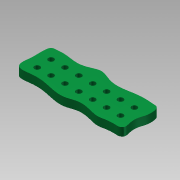
# Autodesk Inventor part: PBD-14 плата
Saved by Autodesk Inventor 2011 (Build 150239000, 239)
## iProperties
Created: 2011-01-23
Part Number: PBD-14 плата
Document SubType Name: Modeling
Designer: Aleirim
Density: 1 g/cm^3
Author: Aleirim
Autodesk Inventor part; units mm, degrees
ref_plane "YZ Plane" through (0, 0, 0) normal (1, 0, 0) x (0, 1, 0)
ref_plane "XZ Plane" through (0, 0, 0) normal (0, 1, 0) x (-1, 0, 0)
ref_plane "XY Plane" through (0, 0, 0) normal (0, 0, 1) x (1, 0, 0)
sketch "Эскиз1" plane through (0, 0, 0) normal (0, 0, 1) x (1, 0, 0)
  spline S0 degree 5 poles (-7.2879, -2.8745) (-6.5517, -2.7913) (-5.2414, -2.7026) (-3.2703, -3.1942) (0.1838, -4.3916) (1.2148, -1.7819) (5.9591, -4.1296) (5.9445, -3.1102) (9.2498, -3.1073) (8.9071, -3.3129) (10.262, -2.8139) (9.4235, -1.6551) (9.4476, 0.385) (10.1818, 0.941) (9.962, 3.5245) (9.2903, 3.5819) (8.0786, 3.5357) (5.6303, 4.053) (1.0268, 1.8567) (-1.261, 5.8579) (-3.117, 2.0115) (-7.1177, 3.7745) (-8.1331, 3.183) (-9.395, 3.43) (-9.6839, 2.8201) (-9.7254, 2.1391) (-9.7847, 0.8422) (-9.6013, -0.2797) (-10.1279, -1.9544) (-9.626, -3.1181) (-8.6028, -3.0516) (-7.7999, -2.9323) (-7.2879, -2.8745) knots 0 0 0 0 0 0 0.061225 0.101586 0.149698 0.194246 0.231169 0.262878 0.289475 0.316265 0.343376 0.374776 0.406255 0.437302 0.468259 0.504653 0.543723 0.588673 0.638889 0.687231 0.727539 0.761442 0.789632 0.813664 0.838456 0.866069 0.896043 0.929673 0.957419 1 1 1 1 1 1
  line L0 (-7.7526, -1.17) -> (-7.7526, -1.37) projected
  line L1 (-7.4863, -1.37) -> (-7.7526, -1.37) projected
  line L2 (-7.4863, -1.37) -> (-7.4863, -1.17) projected
  line L3 (-7.7526, -1.17) -> (-7.4863, -1.17) projected
  circle A0 centre (-7.6194, -1.27) radius 0.5
  line L4 (-7.6194, -1.37) -> (-7.6194, -1.17) construction
  line L5 (-7.7526, -1.27) -> (-7.4863, -1.27) construction
  circle A1 centre (-5.0794, -1.27) radius 0.5
  circle A2 centre (-2.5394, -1.27) radius 0.5
  circle A3 centre (0.0006, -1.27) radius 0.5
  circle A4 centre (2.5406, -1.27) radius 0.5
  circle A5 centre (5.0806, -1.27) radius 0.5
  circle A6 centre (7.6206, -1.27) radius 0.5
  circle A7 centre (-7.6194, 1.27) radius 0.5
  circle A8 centre (-5.0794, 1.27) radius 0.5
  circle A9 centre (-2.5394, 1.27) radius 0.5
  circle A10 centre (0.0006, 1.27) radius 0.5
  circle A11 centre (2.5406, 1.27) radius 0.5
  circle A12 centre (5.0806, 1.27) radius 0.5
  circle A13 centre (7.6206, 1.27) radius 0.5
  point P0 (0, 0)
  point P1 (-0.3454, -3.4271)
  point P2 (2.2796, -2.8745)
  point P3 (5.63, -3.4617)
  point P4 (7.5297, -3.1854)
  point P5 (8.9804, -3.1854)
  point P6 (9.2567, -3.1508)
  point P7 (9.6712, -2.8745)
  point P8 (9.7403, -2.011)
  point P9 (9.6021, 0)
  point P10 (9.982, 1.5466)
  point P11 (9.7403, 3.2045)
  point P12 (9.3258, 3.5154)
  point P13 (8.6004, 3.5845)
  point P14 (6.6317, 3.6536)
  point P15 (1.6579, 3.2391)
  point P16 (-1.3816, 4.0335)
  point P17 (-4.3866, 3.1355)
  point P18 (-7.5988, 3.3772)
  point P19 (-8.7386, 3.3082)
  point P20 (-9.3603, 3.17)
  point P21 (-9.6021, 2.8591)
  point P22 (-9.7057, 2.3065)
  point P23 (-9.7403, 1.2012)
  point P24 (-9.7403, -0.2495)
  point P25 (-9.8439, -1.9419)
  point P26 (-9.2567, -2.8745)
  dimension "d2" = 1
  dimension "d5" = 2.54
  dimension "d8" = 2.54
  constraints: 14 centre point, 6 midpoint, 4 end point, 1 horizontal, 1 vertical, 54 other
  measures "d2" diameter of A0
  measures "d5" distance of A0.centre A1.centre
  measures "d8" distance of A0.centre A7.centre
extrude "Выдавливание2" add sketch "Эскиз1" along normal blind 1.5 contours S0
